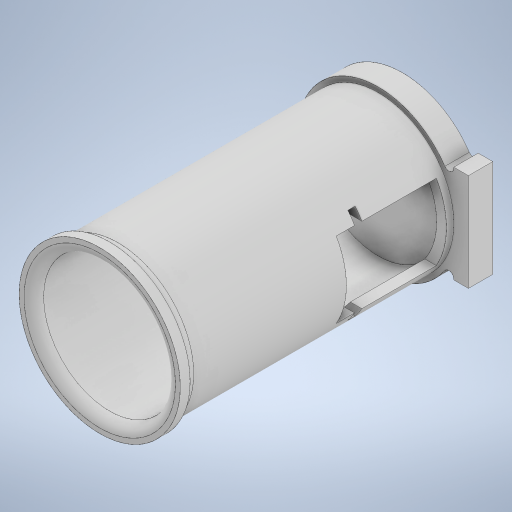
# Autodesk Inventor part: peca1v2
Saved by Autodesk Inventor 2024 (Build 280153000, 153)
## iProperties
Created: 2023-10-22
Part Number: peca1v2
Material: Genérico
Document SubType Name: Modeling
Designer: Daniel
Density: 1 g/cm^3
Appearance: Padrão
Author: Daniel
Autodesk Inventor part; units mm, degrees
ref_plane "XZ Plane" through (0, 0, 0) normal (0, 1, 0) x (-1, 0, 0)
ref_plane "XY Plane" through (0, 0, 0) normal (0, 0, 1) x (1, 0, 0)
sketch "Esboço1" plane through (0, 0, 0) normal (0, 0, 1) x (1, 0, 0)
  circle A0 centre (0, 0) radius 15.5
  dimension "d0" = 31
  constraints: 1 centre point, 1 coincident
  measures "d0" diameter of A0
extrude "Extrusão1" add sketch "Esboço1" along normal blind 2
sketch "Esboço2" plane through (0, 0, 2) normal (0, 0, 1) x (1, 0, 0)
  circle A0 centre (0, 0) radius 15.5 projected
  circle A1 centre (0, 0) radius 13.5
  dimension "d3" = 2
  constraints: 1 centre point
  measures "d3" radial gap between concentric circles of A0 A1
extrude "Extrusão2" add sketch "Esboço2" along normal blind 58
ref_plane "Plano de trabalho4" through (29, 0, 0) normal (1, 0, 0) x (0, 1, 0)
sketch "Esboço5" plane through (29, 0, 0) normal (1, 0, 0) x (0, 1, 0)
  line L0 (-7.75, 27) -> (7.75, 27)
  line L1 (7.75, 27) -> (7.75, 6.5)
  line L2 (7.75, 6.5) -> (-7.75, 6.5)
  line L3 (-7.75, 6.5) -> (-7.75, 27)
  line L4 (-7.75, 27) -> (7.75, 6.5) construction
  line L5 (7.75, 27) -> (-7.75, 6.5) construction
  line L6 (15.5, 0) -> (-15.5, 0) projected
  point P0 (0, 0)
  point P1 (0, 16.75)
  dimension "d15" = 20.5
  dimension "d16" = 15.5
  dimension "d17" = 0
  dimension "d18" = 6.5
  constraints: 12 end point, 2 midpoint, 2 parallel, 1 horizontal, 1 perpendicular
  measures "d15" distance of L0.end L1.end
  measures "d16" distance of L1.end L2.end
  measures "d17" horizontal distance of point (0, 0) point (0, 16.75)
  measures "d18" distance between parallel lines of L6 L2
extrude "Extrusão4" cut sketch "Esboço5" against normal through all
sketch "Esboço7" plane through (0, 0, 60) normal (0, 0, 1) x (1, 0, 0)
  circle A0 centre (0, 0) radius 16.5
  circle A1 centre (0, 0) radius 13.5 projected
  dimension "d28" = 33
  constraints: 1 centre point, 1 coincident
  measures "d28" diameter of A0
extrude "Extrusão6" add sketch "Esboço7" along normal blind 2
fillet "Arredondamento2" radius 2 1 edges at (-13.5, 0, 62)
fillet "Arredondamento3" radius 2 1 edges at (-15.5, 0, 60)
sketch "Sketch8" plane through (0, 0, 0) normal (1, 0, 0) x (0, 1, 0)
  line L0 (-9.75, 21.75) -> (9.75, 21.75)
  line L1 (9.75, 21.75) -> (9.75, 23.25)
  line L2 (9.75, 23.25) -> (-9.75, 23.25)
  line L3 (-9.75, 23.25) -> (-9.75, 21.75)
  line L4 (-7.75, 27) -> (7.75, 27) projected
  line L5 (7.75, 27) -> (7.75, 6.5) projected
  line L6 (-7.75, 6.5) -> (-7.75, 27) projected
  point P0 (0, 0)
  dimension "d37" = 3.75
  dimension "d38" = 1.5
  dimension "d39" = 2
  dimension "d40" = 2
  constraints: 8 end point, 2 parallel, 1 horizontal, 1 perpendicular
  measures "d37" distance between parallel lines of L4 L2
  measures "d38" distance of L0.end L1.end
  measures "d39" distance between parallel lines of L5 L1
  measures "d40" distance between parallel lines of L6 L3
extrude "Extrusion7" cut sketch "Sketch8" along normal mid plane 50 contours L3 L2 L6 L0 | L6 L2 L5 L0 | L5 L2 L1 L0
sketch "Sketch11" plane through (0, 0, 0) normal (0, 0, -1) x (-1, 0, 0)
  line L0 (-18.5, -10) -> (-15.5, -10)
  line L1 (-15.5, -10) -> (-15.5, 10)
  line L2 (-15.5, 10) -> (-18.5, 10)
  line L3 (-18.5, 10) -> (-18.5, -10)
  circle A0 centre (0, 0) radius 16.5 projected
  point P0 (-16.5, 0)
  point P1 (-15.5, 5.6569)
  point P2 (-15.5, -5.6569)
  dimension "d48" = 3
  dimension "d49" = 2
  dimension "d50" = 20
  dimension "d51" = 10
  constraints: 8 end point, 2 parallel, 1 horizontal, 1 perpendicular
  measures "d48" distance of L1.end L2.end
  measures "d49" distance edge to line of A0 L3
  measures "d50" distance of L0.end L1.end
  measures "d51" distance from line of point (0, 0) L0
extrude "Extrusion9" add sketch "Sketch11" against normal blind 5
fillet "Fillet4" radius 1 2 edges at (15.5, 5.6569, 2.5) (15.5, -5.6569, 2.5)
